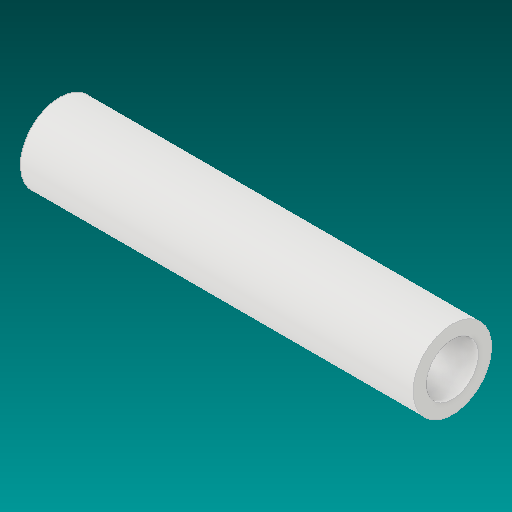
# Autodesk Inventor part: PIJX30-20-150
Saved by Autodesk Inventor 2020 (Build 240168000, 168)
## iProperties
Created: 2022-11-15
Part Number: PIJX30-20-150
Material: Generic
Catalog Web Link: www.cadenas.de
Description: PIJJ, PIJK, PIJM, PIJW, PIJG, PIJT, PIJB, PIJN, PIJF, PIJP, PIJS, PIJX, PIJU-Resin Pipes - ID and OD Surface Finished
Vendor: MISUMI
Document SubType Name: Modeling
Designer: psAdmin
Manufacturer: MISUMI
Mass: 58.9049 g
Surface Area: 243.473 cm^2
Volume: 58.9049 cm^3
Density: 1 g/cm^3
Appearance: PSOLRGB-242-242-242
Category: PARTsolutions
Company: MISUMI
PSOL_IDENT_0: {$CADENAS_DATA/23d-libs/misumi/metric/22_rods_pipes/pijj.prj},259 {VTYP=3D},{NB=PIJX30-20-150},{LINA=
PSOL_IDENT_1: PIJX30-20-150},{NN=PIJJ, PIJK, PIJM, PIJW, PIJG, PIJT, PIJB, PIJN, PIJF, PIJP, PIJS, PIJX, PIJU},{DA
PSOL_IDENT_2: TE=30.06.2021 13:08:38},{GEOMDATE=29.05.2014 00:00:00},{VERSION=},{LINEID=140},{WBVAR=MAT,GRADE,COLO
PSOL_IDENT_3: R,V,L},{WBNUMERIC=V,L}  {NB=PIJX30-20-150},{LINA=PIJX30-20-150},{KT=DUMMY},{PN=PIJX30-20-150},{TYPE=
PSOL_IDENT_4: PIJX},{MAT=ABS},{MATALG= 'P','Polyacetal','MC','MC Nylon','B','Bakelite','F','Fluororesin','PEEK','P
PSOL_IDENT_5: EEK','PPS','PPS','ABS','ABS Resin','UHMWP','Ultra-High-Molecular-Weight-Polyethylene' },{GRADE=S},{G
PSOL_IDENT_6: RADEALG= 'S','Standard' },{COLOR=BE},{COLORALG= 'BE','Beige' },{COL=0.95,0.95,0.95,0.00},{D=30},{V=2
PSOL_IDENT_7: 0},{VALG=16,20,25},{L=150},{LALG=[20:200/1]},{LMIN=20},{LMAX=200}
NB: PIJX30-20-150
NN: PIJJ, PIJK, PIJM, PIJW, PIJG, PIJT, PIJB, PIJN, PIJF, PIJP, PIJS, PIJX, PIJU
NT: Resin Pipes - ID and OD Surface Finished
NBSYN: $PN.
LINA: PIJX30-20-150
CATALOG: Misumi
PN: PIJX30-20-150
MAT: ABS Resin
GRADE: Standard
COLOR: Beige
D: 30
V: 20
L: 150
SUPPLIER: MISUMI
ARTICLENO: PIJX30-20-150
BOMINFO: PIJX30-20-150
CREATOR: CADENAS GmbH
Title: PIJX30-20-150
Author: Cadenas PARTsolutions
Comments: Resin Pipes - ID and OD Surface Finished
Autodesk Inventor part; units mm, degrees
ref_plane "YZ Plane" through (0, 0, 0) normal (1, 0, 0) x (0, 1, 0)
ref_plane "XZ Plane" through (0, 0, 0) normal (0, 1, 0) x (-1, 0, 0)
ref_plane "XY Plane" through (0, 0, 0) normal (0, 0, 1) x (1, 0, 0)
sketch "Sketch_1" plane through (0, 0, 0) normal (0, 0, 1) x (1, 0, 0)
  line L0 (150, 0) -> (0, 0)
  line L1 (0, 10) -> (150, 10)
  line L2 (150, 10) -> (150, 15)
  line L3 (150, 15) -> (0, 15)
  line L4 (0, 15) -> (0, 10)
  constraints: 10 end point
revolve "Revolution1" add sketch "Sketch_1" angle 360 about axis through (150, 0, 0) along (1, 0, 0)
body "Solid1"
